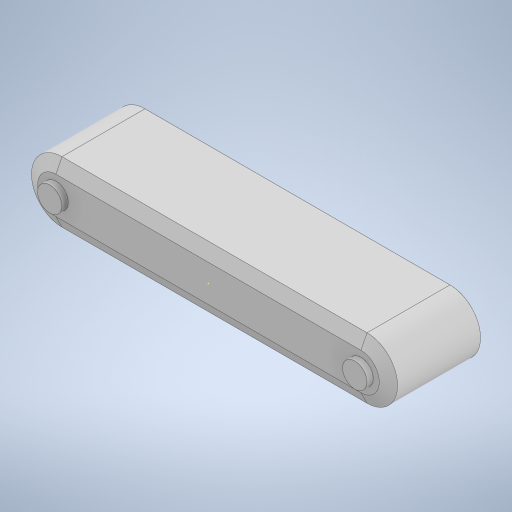
# Autodesk Inventor part: Arm 2 v0.1
Saved by Autodesk Inventor 2023 (Build 270158000, 158)
## iProperties
Created: 2024-06-24
Part Number: Arm 2 v0.1
Material: Generic
Document SubType Name: Modeling
Designer: Swoby
Density: 1 g/cm^3
Appearance: Default
Author: Swoby
Autodesk Inventor part; units mm, degrees
ref_plane "YZ Plane" through (0, 0, 0) normal (1, 0, 0) x (0, 1, 0)
ref_plane "XZ Plane" through (0, 0, 0) normal (0, 1, 0) x (-1, 0, 0)
ref_plane "XY Plane" through (0, 0, 0) normal (0, 0, 1) x (1, 0, 0)
sketch "Sketch1" plane through (0, 0, 0) normal (0, 0, 1) x (1, 0, 0)
  line L0 (-125, 0) -> (125, 0) construction
  line L1 (-125, -25) -> (125, -25)
  line L2 (125, 25) -> (-125, 25)
  arc A0 (-125, 25) -> (-125, -25) centre (-125, 0) ccw
  arc A1 (125, -25) -> (125, 25) centre (125, 0) ccw
  point P0 (0, 0)
  dimension "d0" = 125
  dimension "d1" = 50
  constraints: 8 end point, 4 point on circle, 4 tangent, 2 centre point, 1 horizontal, 1 midpoint, 1 parallel
  measures "d0" distance of point (0, 0) L0.end
  measures "d1" diameter of A1
extrude "Extrusion1" add sketch "Sketch1" along normal blind 78
chamfer "Chamfer1" distance 10 distance2 5 4 edges at (0, -25, 0) (150, 0, 0) (0, 25, 0) (-150, 0, 0) measured on face at (41.6667, -8.3333, 0)
chamfer "Chamfer2" distance 10 distance2 5 4 edges at (0, 25, 78) (-150, 0, 78) (0, -25, 78) (150, 0, 78) measured on face at (41.6667, -8.3333, 78)
sketch "Sketch2" plane through (0, 0, 78) normal (0, 0, 1) x (1, 0, 0)
  point P0 (0, 0)
sketch "Sketch3" plane through (0, 0, 78) normal (0, 0, 1) x (1, 0, 0)
  arc A0 (-125, 15) -> (-125, -15) centre (-125, 0) ccw projected
  arc A1 (125, -15) -> (125, 15) centre (125, 0) ccw projected
  circle A2 centre (-125, 0) radius 10
  circle A3 centre (125, 0) radius 10
  point P0 (0, 0)
  dimension "d10" = 20
  dimension "d11" = 20
  constraints: 2 centre point, 2 coincident
  measures "d10" diameter of A2
  measures "d11" diameter of A3
extrude "Extrusion2" add sketch "Sketch3" along normal blind 5 and the other way blind 83
body "Solid1"
